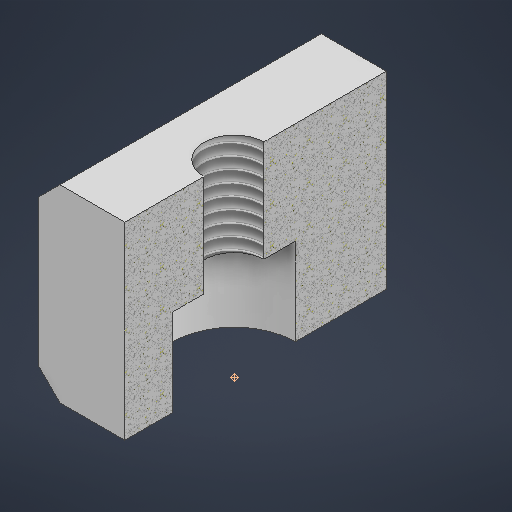
# Autodesk Inventor part: ConTruot
Saved by Autodesk Inventor 2025.4 (Build 294407000, 407)
## iProperties
Created: 2026-05-15
Part Number: ConTruot
Material: Generic
Document SubType Name: Modeling
Designer: VuQuan
Density: 1 g/cm^3
Appearance: Default
Author: VuQuan
Autodesk Inventor part; units mm, degrees
ref_plane "YZ Plane" through (0, 0, 0) normal (1, 0, 0) x (0, 1, 0)
ref_plane "XZ Plane" through (0, 0, 0) normal (0, 1, 0) x (-1, 0, 0)
ref_plane "XY Plane" through (0, 0, 0) normal (0, 0, 1) x (1, 0, 0)
sketch "Sketch1" plane through (0, 0, 0) normal (0, 1, 0) x (-1, 0, 0)
  line L0 (-6, 7.5) -> (6, 7.5)
  line L1 (6, 7.5) -> (6, -10.5)
  line L2 (6, -10.5) -> (-6, -10.5)
  line L3 (-6, -10.5) -> (-6, 7.5)
  circle A0 centre (0, 0) radius 4.25
  point P0 (0, 7.5)
  dimension "d0" = 12
  dimension "d1" = 18
  dimension "d2" = 8.5
  dimension "d3" = 7.5
  constraints: 8 end point, 2 parallel, 1 centre point, 1 coincident, 1 horizontal, 1 midpoint, 1 perpendicular, 1 vertical alignment
  measures "d0" distance of L1.end L2.end
  measures "d1" distance of L0.end L1.end
  measures "d2" diameter of A0
  measures "d3" distance from line of A0.centre L0
extrude "Extrusion1" add sketch "Sketch1" along normal blind 13 contours L0 L1 L2 L3 | A0
extrude "Extrusion2" cut sketch "Sketch1" along normal blind 6 contours A0
chamfer "Chamfer2" distance 1.5 angle 45 4 edges at (6, 13, -1.5) (-6, 13, -1.5) (-6, 0, -1.5) (6, 0, -1.5)
hole "Hole3" at (0, 0, 0) direction (0, 1, 0) diameter 4.134 depth 13 thread size "M5x0.8" class "6H" standard "ISO Metric profile"
body "Solid1"
